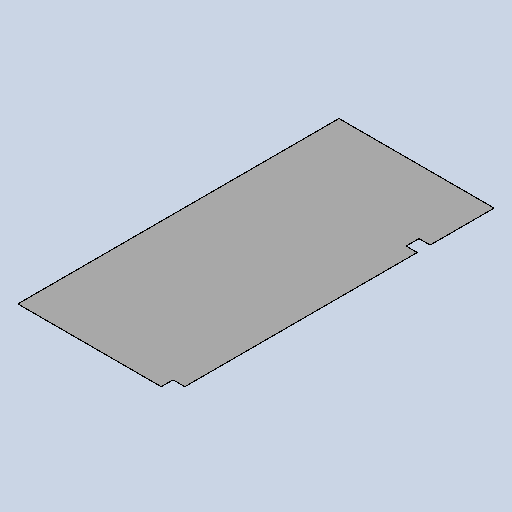
# Autodesk Inventor part: PNS-0111 floor sheet 2
Saved by Autodesk Inventor 2025.1 (Build 291241020, 241B)
## iProperties
Created: 2025-03-10
Part Number: PNS-0111 floor sheet 2
Material: Stainless Steel
Document SubType Name: Sheet Metal
Designer: user
Stock Number: PNS-0111 floor sheet 2
Mass: 72000 g
Surface Area: 90180 cm^2
Volume: 9000 cm^3
Density: 8 g/cm^3
Sheet Metal Rule: AISI304 2mm Die16
Sheet Metal Width: 0.000 mm
Sheet Metal Length: 0.000 mm
Sheet Metal Area: 0.000 mm^2
Appearance: Default
Author: admin
Autodesk Inventor part; units mm, degrees
ref_plane "YZ Plane" through (0, 0, 0) normal (1, 0, 0) x (0, 1, 0)
ref_plane "XZ Plane" through (0, 0, 0) normal (0, 1, 0) x (-1, 0, 0)
ref_plane "XY Plane" through (0, 0, 0) normal (0, 0, 1) x (1, 0, 0)
sketch "Sketch1" plane through (0, 0, 0) normal (0, 0, 1) x (1, 0, 0)
  line L0 (-722.5, -1495) -> (722.5, -1495)
  line L1 (722.5, -1495) -> (722.5, 1495)
  line L2 (722.5, 1495) -> (-722.5, 1495)
  line L3 (-722.5, 1495) -> (-722.5, -1495)
  line L4 (-722.5, -1495) -> (722.5, 1495) construction
  line L5 (722.5, -1495) -> (-722.5, 1495) construction
  line L6 (722.5, -1385) -> (612.5, -1385)
  line L7 (612.5, -1385) -> (612.5, -1495)
  line L8 (722.5, 899) -> (618.5, 899)
  line L9 (618.5, 899) -> (618.5, 779)
  line L10 (618.5, 779) -> (722.5, 779)
  line L11 (722.5, 779) -> (722.5, 899)
  point P0 (0, 0)
  point P1 (722.5, 779)
  dimension "d154" = 1445
  dimension "d155" = 2990
  dimension "d157" = 110
  dimension "d159" = 120
  dimension "d160" = 596
  dimension "d161" = 104
  measures "d154" distance of L1.end L2.end
  measures "d155" distance of L0.end L1.end
  measures "d157" distance of L6.start L6.end
  measures "d159" distance of L8.end L9.end
  measures "d160" distance between parallel lines of L8 L2
  measures "d161" distance of L9.end L10.end
extrude "Plate5" add sketch "Sketch1" along normal blind 2 contours L3 L2 L1 L8 L9 L10 L6 L7 L0
fillet "Corner Round1" radius 15 1 edges at (612.5, -1385, 1)
body "Solid3"
